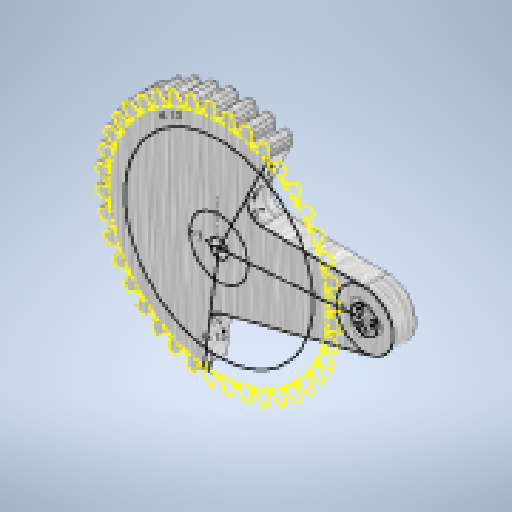
# Autodesk Inventor part: 最終段m2z40
Saved by Autodesk Inventor 2023 (Build 270158030, 158C)
## iProperties
Created: 2022-03-13
Part Number: 最終段m2z40
Material: アルミニウム 7075
Document SubType Name: Modeling
Designer: acps
Density: 2.81 g/cm^3
Appearance: サテン - ブラシ仕上げ 重厚
Author: acps
Autodesk Inventor part; units mm, degrees
(part 1 of 2)
ref_plane "YZ Plane" through (0, 0, 0) normal (1, 0, 0) x (0, 1, 0)
ref_plane "XZ Plane" through (0, 0, 0) normal (0, 1, 0) x (-1, 0, 0)
ref_plane "XY Plane" through (0, 0, 0) normal (0, 0, 1) x (1, 0, 0)
sketch "Sketch1" plane through (0, 0, 0) normal (0, 0, 1) x (1, 0, 0)
  arc A0 (0.9701, 39.1647) -> (0.7425, 38.3328) centre (9.8386, 36.2911) ccw
  arc A1 (1.4107, 40.3306) -> (0.9701, 39.1647) centre (13.2368, 35.1958) ccw
  arc A2 (2.1934, 41.9015) -> (1.4107, 40.3306) centre (16.718, 33.6843) ccw
  arc A3 (-5.1685, 38.8343) -> (-5.2632, 37.977) centre (4.0403, 37.3834) ccw
  arc A4 (-4.913, 40.0655) -> (-5.1685, 38.8343) centre (7.568, 36.8332) ccw
  arc A5 (-4.3885, 41.7288) -> (-4.913, 40.0655) centre (11.2428, 35.8848) ccw
  arc A6 (-11.1799, 37.5477) -> (-11.1393, 36.6861) centre (-1.8575, 37.5552) ccw
  arc A7 (-11.1212, 38.7926) -> (-11.1799, 37.5477) centre (1.7129, 37.5636) ccw
  arc A8 (-10.8623, 40.5285) -> (-11.1212, 38.7926) centre (5.4908, 37.2018) ccw
  arc A9 (-16.916, 35.3365) -> (-16.7411, 34.4919) centre (-7.7096, 36.8023) ccw
  arc A10 (-17.0535, 36.5863) -> (-16.916, 35.3365) centre (-4.1845, 37.3691) ccw
  arc A11 (-17.0686, 38.3303) -> (-17.0535, 36.5863) centre (-0.3965, 37.6027) ccw
  arc A12 (-22.2356, 32.2552) -> (-21.9307, 31.4483) centre (-13.3718, 35.1431) ccw
  arc A13 (-22.5669, 33.4681) -> (-22.2356, 32.2552) centre (-9.9788, 36.2544) ccw
  arc A14 (-22.8546, 35.1883) -> (-22.5669, 33.4681) centre (-6.2739, 37.0778) ccw
  arc A15 (-27.0076, 28.3796) -> (-26.5803, 27.6304) centre (-18.7048, 32.6187) ccw
  arc A16 (-27.5246, 29.5259) -> (-27.0076, 28.3796) centre (-15.5273, 34.247) ccw
  arc A17 (-28.0779, 31.1798) -> (-27.5246, 29.5259) centre (-11.9969, 35.6398) ccw
  arc A18 (-31.1147, 23.8053) -> (-30.5755, 23.1322) centre (-23.5772, 29.291) ccw
  arc A19 (-31.8046, 24.8565) -> (-31.1147, 23.8053) centre (-20.6936, 31.3964) ccw
  arc A20 (-32.6098, 26.4036) -> (-31.8046, 24.8565) centre (-17.4245, 33.3243) ccw
  arc A21 (-34.4556, 18.6448) -> (-33.8177, 18.0643) centre (-27.869, 25.2421) ccw
  arc A22 (-35.3014, 19.5752) -> (-34.4556, 18.6448) centre (-25.3503, 27.7726) ccw
  arc A23 (-36.3388, 20.9772) -> (-35.3014, 19.5752) centre (-22.4231, 30.1882) ccw
  arc A24 (-36.9365, 13.0169) -> (-36.2272, 12.5517) centre (-31.4746, 20.5717) ccw
  arc A25 (-37.9291, 13.8118) -> (-36.9365, 13.0169) centre (-29.3828, 23.4651) ccw
  arc A26 (-39.1729, 15.0343) -> (-37.9291, 13.8118) centre (-26.8695, 26.3088) ccw
  arc A27 (-38.5308, 7.0849) -> (-37.7447, 6.73) centre (-34.3052, 15.3947) ccw
  arc A28 (-39.6227, 7.7084) -> (-38.5308, 7.0849) centre (-32.6918, 18.5797) ccw
  arc A29 (-41.0425, 8.7212) -> (-39.6227, 7.7084) centre (-30.6543, 21.7816) ccw
  arc A30 (-39.1647, 0.9701) -> (-38.3328, 0.7425) centre (-36.2911, 9.8386) ccw
  arc A31 (-40.3306, 1.4107) -> (-39.1647, 0.9701) centre (-35.1958, 13.2368) ccw
  arc A32 (-41.9015, 2.1934) -> (-40.3306, 1.4107) centre (-33.6843, 16.718) ccw
  arc A33 (-38.8343, -5.1685) -> (-37.977, -5.2632) centre (-37.3834, 4.0403) ccw
  arc A34 (-40.0655, -4.913) -> (-38.8343, -5.1685) centre (-36.8332, 7.568) ccw
  arc A35 (-41.7288, -4.3885) -> (-40.0655, -4.913) centre (-35.8848, 11.2428) ccw
  arc A36 (-37.5477, -11.1799) -> (-36.6861, -11.1393) centre (-37.5552, -1.8575) ccw
  arc A37 (-38.7926, -11.1212) -> (-37.5477, -11.1799) centre (-37.5636, 1.7129) ccw
  arc A38 (-40.5285, -10.8623) -> (-38.7926, -11.1212) centre (-37.2018, 5.4908) ccw
  arc A39 (-35.3365, -16.916) -> (-34.4919, -16.7411) centre (-36.8023, -7.7096) ccw
  arc A40 (-36.5863, -17.0535) -> (-35.3365, -16.916) centre (-37.3691, -4.1845) ccw
  arc A41 (-38.3303, -17.0686) -> (-36.5863, -17.0535) centre (-37.6027, -0.3965) ccw
  arc A42 (-32.2552, -22.2356) -> (-31.4483, -21.9307) centre (-35.1431, -13.3718) ccw
  arc A43 (-33.4681, -22.5669) -> (-32.2552, -22.2356) centre (-36.2544, -9.9788) ccw
  arc A44 (-35.1883, -22.8546) -> (-33.4681, -22.5669) centre (-37.0778, -6.2739) ccw
  arc A45 (-28.3796, -27.0076) -> (-27.6304, -26.5803) centre (-32.6187, -18.7048) ccw
  arc A46 (-29.5259, -27.5246) -> (-28.3796, -27.0076) centre (-34.247, -15.5273) ccw
  arc A47 (-31.1798, -28.0779) -> (-29.5259, -27.5246) centre (-35.6398, -11.9969) ccw
  arc A48 (-23.8053, -31.1147) -> (-23.1322, -30.5754) centre (-29.291, -23.5771) ccw
  arc A49 (-24.8565, -31.8046) -> (-23.8053, -31.1147) centre (-31.3964, -20.6936) ccw
  arc A50 (-26.4036, -32.6098) -> (-24.8565, -31.8046) centre (-33.3243, -17.4245) ccw
  arc A51 (-18.6448, -34.4556) -> (-18.0643, -33.8177) centre (-25.2421, -27.869) ccw
  arc A52 (-19.5752, -35.3014) -> (-18.6448, -34.4556) centre (-27.7726, -25.3503) ccw
  arc A53 (-20.9772, -36.3388) -> (-19.5752, -35.3014) centre (-30.1882, -22.4231) ccw
  arc A54 (-13.0252, -36.9481) -> (-12.5517, -36.2272) centre (-20.5717, -31.4746) ccw
  arc A55 (-13.8118, -37.9291) -> (-13.0252, -36.9481) centre (-23.4651, -29.3828) ccw
  arc A56 (-15.0343, -39.1729) -> (-13.8118, -37.9291) centre (-26.3088, -26.8695) ccw
  arc A57 (-7.0849, -38.5308) -> (-6.73, -37.7447) centre (-15.3947, -34.3052) ccw
  arc A58 (-7.7084, -39.6227) -> (-7.0849, -38.5308) centre (-18.5797, -32.6918) ccw
  arc A59 (-8.7212, -41.0425) -> (-7.7084, -39.6227) centre (-21.7816, -30.6543) ccw
  arc A60 (-0.9701, -39.1647) -> (-0.7425, -38.3328) centre (-9.8386, -36.2911) ccw
  arc A61 (-1.4151, -40.3408) -> (-0.9701, -39.1647) centre (-13.2368, -35.1958) ccw
  arc A62 (-2.1934, -41.9015) -> (-1.4151, -40.3408) centre (-16.718, -33.6843) ccw
  arc A63 (5.1685, -38.8343) -> (5.2632, -37.977) centre (-4.0403, -37.3834) ccw
  arc A64 (4.913, -40.0655) -> (5.1685, -38.8343) centre (-7.568, -36.8332) ccw
  arc A65 (4.3885, -41.7288) -> (4.913, -40.0655) centre (-11.2428, -35.8848) ccw
  arc A66 (11.1799, -37.5477) -> (11.1393, -36.6861) centre (1.8575, -37.5552) ccw
  arc A67 (11.1201, -38.8036) -> (11.1799, -37.5477) centre (-1.7129, -37.5636) ccw
  arc A68 (10.8623, -40.5285) -> (11.1201, -38.8036) centre (-5.4908, -37.2018) ccw
  arc A69 (16.916, -35.3365) -> (16.7411, -34.4919) centre (7.7096, -36.8023) ccw
  arc A70 (17.0535, -36.5863) -> (16.916, -35.3365) centre (4.1845, -37.3691) ccw
  arc A71 (17.0686, -38.3303) -> (17.0535, -36.5863) centre (0.3965, -37.6027) ccw
  arc A72 (22.2356, -32.2552) -> (21.9307, -31.4483) centre (13.3718, -35.1431) ccw
  arc A73 (22.5669, -33.4681) -> (22.2356, -32.2552) centre (9.9788, -36.2544) ccw
  arc A74 (22.8546, -35.1883) -> (22.5669, -33.4681) centre (6.2739, -37.0778) ccw
  arc A75 (27.0076, -28.3796) -> (26.5803, -27.6304) centre (18.7048, -32.6187) ccw
  arc A76 (27.5246, -29.5259) -> (27.0076, -28.3796) centre (15.5273, -34.247) ccw
  arc A77 (28.0779, -31.1798) -> (27.5246, -29.5259) centre (11.9969, -35.6398) ccw
  arc A78 (31.1147, -23.8053) -> (30.5755, -23.1322) centre (23.5772, -29.291) ccw
  arc A79 (31.8046, -24.8565) -> (31.1147, -23.8053) centre (20.6936, -31.3964) ccw
  arc A80 (32.6098, -26.4036) -> (31.8046, -24.8565) centre (17.4245, -33.3243) ccw
  arc A81 (34.4556, -18.6448) -> (33.8177, -18.0643) centre (27.869, -25.2421) ccw
  arc A82 (35.3014, -19.5752) -> (34.4556, -18.6448) centre (25.3503, -27.7726) ccw
  arc A83 (36.3388, -20.9772) -> (35.3014, -19.5752) centre (22.4231, -30.1882) ccw
  arc A84 (36.9481, -13.0252) -> (36.2272, -12.5517) centre (31.4746, -20.5717) ccw
  arc A85 (37.9291, -13.8118) -> (36.9481, -13.0252) centre (29.3828, -23.4651) ccw
  arc A86 (39.1729, -15.0343) -> (37.9291, -13.8118) centre (26.8695, -26.3088) ccw
  arc A87 (38.5308, -7.0849) -> (37.7447, -6.73) centre (34.3052, -15.3947) ccw
  arc A88 (39.6227, -7.7084) -> (38.5308, -7.0849) centre (32.6918, -18.5797) ccw
  arc A89 (41.0425, -8.7212) -> (39.6227, -7.7084) centre (30.6543, -21.7816) ccw
  arc A90 (39.1647, -0.9701) -> (38.3328, -0.7425) centre (36.2911, -9.8386) ccw
  arc A91 (40.3408, -1.4151) -> (39.1647, -0.9701) centre (35.1958, -13.2368) ccw
  arc A92 (41.9015, -2.1934) -> (40.3408, -1.4151) centre (33.6843, -16.718) ccw
  arc A93 (38.8343, 5.1685) -> (37.977, 5.2632) centre (37.3834, -4.0403) ccw
  arc A94 (40.0655, 4.913) -> (38.8343, 5.1685) centre (36.8332, -7.568) ccw
  arc A95 (41.7288, 4.3885) -> (40.0655, 4.913) centre (35.8848, -11.2428) ccw
  arc A96 (37.5477, 11.1799) -> (36.6861, 11.1393) centre (37.5552, 1.8575) ccw
  arc A97 (38.8036, 11.1201) -> (37.5477, 11.1799) centre (37.5636, -1.7129) ccw
  arc A98 (40.5285, 10.8623) -> (38.8036, 11.1201) centre (37.2018, -5.4908) ccw
  arc A99 (35.3365, 16.916) -> (34.4919, 16.7411) centre (36.8023, 7.7096) ccw
  arc A100 (36.5863, 17.0535) -> (35.3365, 16.916) centre (37.3691, 4.1845) ccw
  arc A101 (38.3303, 17.0686) -> (36.5863, 17.0535) centre (37.6027, 0.3965) ccw
  arc A102 (32.2552, 22.2356) -> (31.4483, 21.9307) centre (35.1431, 13.3718) ccw
  arc A103 (33.4681, 22.5669) -> (32.2552, 22.2356) centre (36.2544, 9.9788) ccw
  arc A104 (35.1883, 22.8546) -> (33.4681, 22.5669) centre (37.0778, 6.2739) ccw
  arc A105 (28.3796, 27.0076) -> (27.6304, 26.5803) centre (32.6187, 18.7048) ccw
  arc A106 (29.5259, 27.5246) -> (28.3796, 27.0076) centre (34.247, 15.5273) ccw
  arc A107 (31.1798, 28.0779) -> (29.5259, 27.5246) centre (35.6398, 11.9969) ccw
  arc A108 (23.8053, 31.1147) -> (23.1322, 30.5755) centre (29.291, 23.5772) ccw
  arc A109 (24.8565, 31.8046) -> (23.8053, 31.1147) centre (31.3964, 20.6936) ccw
  arc A110 (26.4036, 32.6098) -> (24.8565, 31.8046) centre (33.3243, 17.4245) ccw
  arc A111 (18.6448, 34.4556) -> (18.0643, 33.8177) centre (25.2421, 27.869) ccw
  arc A112 (19.5752, 35.3014) -> (18.6448, 34.4556) centre (27.7726, 25.3503) ccw
  arc A113 (20.9772, 36.3388) -> (19.5752, 35.3014) centre (30.1882, 22.4231) ccw
  arc A114 (13.0252, 36.9481) -> (12.5517, 36.2272) centre (20.5717, 31.4746) ccw
  arc A115 (13.8118, 37.9291) -> (13.0252, 36.9481) centre (23.4651, 29.3828) ccw
  arc A116 (15.0343, 39.1729) -> (13.8118, 37.9291) centre (26.3088, 26.8695) ccw
  arc A117 (7.0849, 38.5308) -> (6.73, 37.7447) centre (15.3947, 34.3052) ccw
  arc A118 (7.7084, 39.6227) -> (7.0849, 38.5308) centre (18.5797, 32.6918) ccw
  arc A119 (8.7212, 41.0425) -> (7.7084, 39.6227) centre (21.7816, 30.6543) ccw
  arc A120 (-0.7425, 38.3328) -> (-0.9657, 39.1511) centre (-9.8386, 36.2911) ccw
  arc A121 (-0.9657, 39.1511) -> (-1.4151, 40.3408) centre (-13.2368, 35.1958) ccw
  arc A122 (-1.4151, 40.3408) -> (-2.1934, 41.9015) centre (-16.718, 33.6843) ccw
  arc A123 (-6.73, 37.7447) -> (-7.0849, 38.5308) centre (-15.3947, 34.3052) ccw
  arc A124 (-7.0849, 38.5308) -> (-7.7084, 39.6227) centre (-18.5797, 32.6918) ccw
  arc A125 (-7.7084, 39.6227) -> (-8.7212, 41.0425) centre (-21.7816, 30.6543) ccw
  arc A126 (-12.5517, 36.2272) -> (-13.0252, 36.9481) centre (-20.5717, 31.4746) ccw
  arc A127 (-13.0252, 36.9481) -> (-13.8118, 37.9291) centre (-23.4651, 29.3828) ccw
  arc A128 (-13.8118, 37.9291) -> (-15.0343, 39.1729) centre (-26.3088, 26.8695) ccw
  arc A129 (-18.0643, 33.8177) -> (-18.6448, 34.4556) centre (-25.2421, 27.869) ccw
  arc A130 (-18.6448, 34.4556) -> (-19.5752, 35.3014) centre (-27.7726, 25.3503) ccw
  arc A131 (-19.5752, 35.3014) -> (-20.9772, 36.3388) centre (-30.1882, 22.4231) ccw
  arc A132 (-23.1322, 30.5755) -> (-23.8053, 31.1147) centre (-29.291, 23.5772) ccw
  arc A133 (-23.8053, 31.1147) -> (-24.8565, 31.8046) centre (-31.3964, 20.6936) ccw
  arc A134 (-24.8565, 31.8046) -> (-26.4036, 32.6098) centre (-33.3243, 17.4245) ccw
  arc A135 (-27.6304, 26.5803) -> (-28.3796, 27.0076) centre (-32.6187, 18.7048) ccw
  arc A136 (-28.3796, 27.0076) -> (-29.5259, 27.5246) centre (-34.247, 15.5273) ccw
  arc A137 (-29.5259, 27.5246) -> (-31.1798, 28.0779) centre (-35.6398, 11.9969) ccw
  arc A138 (-31.4483, 21.9307) -> (-32.2552, 22.2356) centre (-35.1431, 13.3718) ccw
  arc A139 (-32.2552, 22.2356) -> (-33.4681, 22.5669) centre (-36.2544, 9.9788) ccw
  arc A140 (-33.4681, 22.5669) -> (-35.1883, 22.8546) centre (-37.0778, 6.2739) ccw
  arc A141 (-34.4919, 16.7411) -> (-35.3365, 16.916) centre (-36.8023, 7.7096) ccw
  arc A142 (-35.3365, 16.916) -> (-36.5863, 17.0535) centre (-37.3691, 4.1845) ccw
  arc A143 (-36.5863, 17.0535) -> (-38.3303, 17.0686) centre (-37.6027, 0.3965) ccw
  arc A144 (-36.6861, 11.1393) -> (-37.5477, 11.1799) centre (-37.5552, 1.8575) ccw
  arc A145 (-37.5477, 11.1799) -> (-38.8036, 11.1201) centre (-37.5636, -1.7129) ccw
  arc A146 (-38.8036, 11.1201) -> (-40.5285, 10.8623) centre (-37.2018, -5.4908) ccw
  arc A147 (-37.977, 5.2632) -> (-38.8343, 5.1685) centre (-37.3834, -4.0403) ccw
  arc A148 (-38.8343, 5.1685) -> (-40.0655, 4.913) centre (-36.8332, -7.568) ccw
  arc A149 (-40.0655, 4.913) -> (-41.7288, 4.3885) centre (-35.8848, -11.2428) ccw
  arc A150 (-38.3328, -0.7425) -> (-39.1647, -0.9701) centre (-36.2911, -9.8386) ccw
  arc A151 (-39.1647, -0.9701) -> (-40.3306, -1.4107) centre (-35.1958, -13.2368) ccw
  arc A152 (-40.3306, -1.4107) -> (-41.9015, -2.1934) centre (-33.6843, -16.718) ccw
  arc A153 (-37.7447, -6.73) -> (-38.5308, -7.0849) centre (-34.3052, -15.3947) ccw
  arc A154 (-38.5308, -7.0849) -> (-39.6227, -7.7084) centre (-32.6918, -18.5797) ccw
  arc A155 (-39.6227, -7.7084) -> (-41.0425, -8.7212) centre (-30.6543, -21.7816) ccw
  arc A156 (-36.2272, -12.5517) -> (-36.9481, -13.0252) centre (-31.4746, -20.5717) ccw
  arc A157 (-36.9481, -13.0252) -> (-37.9291, -13.8118) centre (-29.3828, -23.4651) ccw
  arc A158 (-37.9291, -13.8118) -> (-39.1729, -15.0343) centre (-26.8695, -26.3088) ccw
  arc A159 (-33.8177, -18.0643) -> (-34.4556, -18.6448) centre (-27.869, -25.2421) ccw
  arc A160 (-34.4556, -18.6448) -> (-35.3014, -19.5752) centre (-25.3503, -27.7726) ccw
  arc A161 (-35.3014, -19.5752) -> (-36.3388, -20.9772) centre (-22.4231, -30.1882) ccw
  arc A162 (-30.5754, -23.1322) -> (-31.1147, -23.8053) centre (-23.5771, -29.291) ccw
  arc A163 (-31.1147, -23.8053) -> (-31.8046, -24.8565) centre (-20.6936, -31.3964) ccw
  arc A164 (-31.8046, -24.8565) -> (-32.6098, -26.4036) centre (-17.4245, -33.3243) ccw
  arc A165 (-26.5803, -27.6304) -> (-27.0076, -28.3796) centre (-18.7048, -32.6187) ccw
  arc A166 (-27.0076, -28.3796) -> (-27.5246, -29.5259) centre (-15.5273, -34.247) ccw
  arc A167 (-27.5246, -29.5259) -> (-28.0779, -31.1798) centre (-11.9969, -35.6398) ccw
  arc A168 (-21.9307, -31.4483) -> (-22.2356, -32.2552) centre (-13.3718, -35.1431) ccw
  arc A169 (-22.2356, -32.2552) -> (-22.5669, -33.4681) centre (-9.9788, -36.2544) ccw
  arc A170 (-22.5669, -33.4681) -> (-22.8546, -35.1883) centre (-6.2739, -37.0778) ccw
  arc A171 (-16.7411, -34.4919) -> (-16.916, -35.3365) centre (-7.7096, -36.8023) ccw
  arc A172 (-16.916, -35.3365) -> (-17.0535, -36.5863) centre (-4.1845, -37.3691) ccw
  arc A173 (-17.0535, -36.5863) -> (-17.0686, -38.3303) centre (-0.3965, -37.6027) ccw
  arc A174 (-11.1393, -36.6861) -> (-11.1799, -37.5477) centre (-1.8575, -37.5552) ccw
  arc A175 (-11.1799, -37.5477) -> (-11.1201, -38.8036) centre (1.7129, -37.5636) ccw
  arc A176 (-11.1201, -38.8036) -> (-10.8623, -40.5285) centre (5.4908, -37.2018) ccw
  arc A177 (-5.2632, -37.977) -> (-5.1685, -38.8343) centre (4.0403, -37.3834) ccw
  arc A178 (-5.1685, -38.8343) -> (-4.913, -40.0655) centre (7.568, -36.8332) ccw
  arc A179 (-4.913, -40.0655) -> (-4.3885, -41.7288) centre (11.2428, -35.8848) ccw
  arc A180 (0.7425, -38.3328) -> (0.9701, -39.1647) centre (9.8386, -36.2911) ccw
  arc A181 (0.9701, -39.1647) -> (1.4151, -40.3408) centre (13.2368, -35.1958) ccw
  arc A182 (1.4151, -40.3408) -> (2.1934, -41.9015) centre (16.718, -33.6843) ccw
  arc A183 (6.73, -37.7447) -> (7.0849, -38.5308) centre (15.3947, -34.3052) ccw
  arc A184 (7.0849, -38.5308) -> (7.7084, -39.6227) centre (18.5797, -32.6918) ccw
  arc A185 (7.7084, -39.6227) -> (8.7212, -41.0425) centre (21.7816, -30.6543) ccw
  arc A186 (12.5517, -36.2272) -> (13.0252, -36.9481) centre (20.5717, -31.4746) ccw
  arc A187 (13.0252, -36.9481) -> (13.8118, -37.9291) centre (23.4651, -29.3828) ccw
  arc A188 (13.8118, -37.9291) -> (15.0343, -39.1729) centre (26.3088, -26.8695) ccw
  arc A189 (18.0643, -33.8177) -> (18.6448, -34.4556) centre (25.2421, -27.869) ccw
  arc A190 (18.6448, -34.4556) -> (19.5752, -35.3014) centre (27.7726, -25.3503) ccw
  arc A191 (19.5752, -35.3014) -> (20.9772, -36.3388) centre (30.1882, -22.4231) ccw
  arc A192 (23.1322, -30.5755) -> (23.8053, -31.1147) centre (29.291, -23.5772) ccw
  arc A193 (23.8053, -31.1147) -> (24.8565, -31.8046) centre (31.3964, -20.6936) ccw
  arc A194 (24.8565, -31.8046) -> (26.4036, -32.6098) centre (33.3243, -17.4245) ccw
  arc A195 (27.6304, -26.5803) -> (28.3796, -27.0076) centre (32.6187, -18.7048) ccw
  arc A196 (28.3796, -27.0076) -> (29.5259, -27.5246) centre (34.247, -15.5273) ccw
  arc A197 (29.5259, -27.5246) -> (31.1798, -28.0779) centre (35.6398, -11.9969) ccw
  arc A198 (31.4483, -21.9307) -> (32.2552, -22.2356) centre (35.1431, -13.3718) ccw
  arc A199 (32.2552, -22.2356) -> (33.4681, -22.5669) centre (36.2544, -9.9788) ccw
  arc A200 (33.4681, -22.5669) -> (35.1883, -22.8546) centre (37.0778, -6.2739) ccw
  arc A201 (34.4919, -16.7411) -> (35.3365, -16.916) centre (36.8023, -7.7096) ccw
  arc A202 (35.3365, -16.916) -> (36.5863, -17.0535) centre (37.3691, -4.1845) ccw
  arc A203 (36.5863, -17.0535) -> (38.3303, -17.0686) centre (37.6027, -0.3965) ccw
  arc A204 (36.6861, -11.1393) -> (37.5477, -11.1799) centre (37.5552, -1.8575) ccw
  arc A205 (37.5477, -11.1799) -> (38.8036, -11.1201) centre (37.5636, 1.7129) ccw
  arc A206 (38.8036, -11.1201) -> (40.5285, -10.8623) centre (37.2018, 5.4908) ccw
  arc A207 (37.977, -5.2632) -> (38.8343, -5.1685) centre (37.3834, 4.0403) ccw
  arc A208 (38.8343, -5.1685) -> (40.0655, -4.913) centre (36.8332, 7.568) ccw
  arc A209 (40.0655, -4.913) -> (41.7288, -4.3885) centre (35.8848, 11.2428) ccw
  arc A210 (38.3328, 0.7425) -> (39.1647, 0.9701) centre (36.2911, 9.8386) ccw
  arc A211 (39.1647, 0.9701) -> (40.3306, 1.4107) centre (35.1958, 13.2368) ccw
  arc A212 (40.3306, 1.4107) -> (41.9015, 2.1934) centre (33.6843, 16.718) ccw
  arc A213 (37.7447, 6.73) -> (38.5308, 7.0849) centre (34.3052, 15.3947) ccw
  arc A214 (38.5308, 7.0849) -> (39.6227, 7.7084) centre (32.6918, 18.5797) ccw
  arc A215 (39.6227, 7.7084) -> (41.0425, 8.7212) centre (30.6543, 21.7816) ccw
  arc A216 (36.2272, 12.5517) -> (36.9481, 13.0252) centre (31.4746, 20.5717) ccw
  arc A217 (36.9481, 13.0252) -> (37.9207, 13.8045) centre (29.3828, 23.4651) ccw
  arc A218 (37.9207, 13.8045) -> (39.1729, 15.0343) centre (26.8695, 26.3088) ccw
  arc A219 (33.8177, 18.0643) -> (34.4556, 18.6448) centre (27.869, 25.2421) ccw
  arc A220 (34.4556, 18.6448) -> (35.3014, 19.5752) centre (25.3503, 27.7726) ccw
  arc A221 (35.3014, 19.5752) -> (36.3388, 20.9772) centre (22.4231, 30.1882) ccw
  arc A222 (30.5755, 23.1322) -> (31.1147, 23.8053) centre (23.5772, 29.291) ccw
  arc A223 (31.1147, 23.8053) -> (31.8046, 24.8565) centre (20.6936, 31.3964) ccw
  arc A224 (31.8046, 24.8565) -> (32.6098, 26.4036) centre (17.4245, 33.3243) ccw
  arc A225 (26.5803, 27.6304) -> (27.0076, 28.3796) centre (18.7048, 32.6187) ccw
  arc A226 (27.0076, 28.3796) -> (27.5246, 29.5259) centre (15.5273, 34.247) ccw
  arc A227 (27.5246, 29.5259) -> (28.0779, 31.1798) centre (11.9969, 35.6398) ccw
  arc A228 (21.9307, 31.4483) -> (22.2356, 32.2552) centre (13.3718, 35.1431) ccw
  arc A229 (22.2356, 32.2552) -> (22.5669, 33.4681) centre (9.9788, 36.2544) ccw
  arc A230 (22.5669, 33.4681) -> (22.8546, 35.1883) centre (6.2739, 37.0778) ccw
  arc A231 (16.7411, 34.4919) -> (16.916, 35.3365) centre (7.7096, 36.8023) ccw
  arc A232 (16.916, 35.3365) -> (17.0535, 36.5863) centre (4.1845, 37.3691) ccw
  arc A233 (17.0535, 36.5863) -> (17.0686, 38.3303) centre (0.3965, 37.6027) ccw
  arc A234 (11.1393, 36.6861) -> (11.1799, 37.5477) centre (1.8575, 37.5552) ccw
  arc A235 (11.1799, 37.5477) -> (11.1201, 38.8036) centre (-1.7129, 37.5636) ccw
  arc A236 (11.1201, 38.8036) -> (10.8623, 40.5285) centre (-5.4908, 37.2018) ccw
  arc A237 (5.2632, 37.977) -> (5.1685, 38.8343) centre (-4.0403, 37.3834) ccw
  arc A238 (5.1685, 38.8343) -> (4.9158, 40.0547) centre (-7.568, 36.8332) ccw
  arc A239 (4.9158, 40.0547) -> (4.3885, 41.7288) centre (-11.2428, 35.8848) ccw
  arc A240 (0.7425, 38.3328) -> (-0.7425, 38.3328) centre (0, 0) ccw
  arc A241 (-5.2632, 37.977) -> (-6.73, 37.7447) centre (0, 0) ccw
  arc A242 (-11.1393, 36.6861) -> (-12.5517, 36.2272) centre (0, 0) ccw
  arc A243 (-16.7411, 34.4919) -> (-18.0643, 33.8177) centre (0, 0) ccw
  arc A244 (-21.9307, 31.4483) -> (-23.1322, 30.5755) centre (0, 0) ccw
  arc A245 (-26.5803, 27.6304) -> (-27.6304, 26.5803) centre (0, 0) ccw
  arc A246 (-30.5755, 23.1322) -> (-31.4483, 21.9307) centre (0, 0) ccw
  arc A247 (-33.8177, 18.0643) -> (-34.4919, 16.7411) centre (0, 0) ccw
  arc A248 (-36.2272, 12.5517) -> (-36.6861, 11.1393) centre (0, 0) ccw
  arc A249 (-37.7447, 6.73) -> (-37.977, 5.2632) centre (0, 0) ccw
  arc A250 (-38.3328, 0.7425) -> (-38.3328, -0.7425) centre (0, 0) ccw
  arc A251 (-37.977, -5.2632) -> (-37.7447, -6.73) centre (0, 0) ccw
  arc A252 (-36.6861, -11.1393) -> (-36.2272, -12.5517) centre (0, 0) ccw
  arc A253 (-34.4919, -16.7411) -> (-33.8177, -18.0643) centre (0, 0) ccw
  arc A254 (-31.4483, -21.9307) -> (-30.5754, -23.1322) centre (0, 0) ccw
  arc A255 (-27.6304, -26.5803) -> (-26.5803, -27.6304) centre (0, 0) ccw
  arc A256 (-23.1322, -30.5754) -> (-21.9307, -31.4483) centre (0, 0) ccw
  arc A257 (-18.0643, -33.8177) -> (-16.7411, -34.4919) centre (0, 0) ccw
  arc A258 (-12.5517, -36.2272) -> (-11.1393, -36.6861) centre (0, 0) ccw
  arc A259 (-6.73, -37.7447) -> (-5.2632, -37.977) centre (0, 0) ccw
  arc A260 (-0.7425, -38.3328) -> (0.7425, -38.3328) centre (0, 0) ccw
  arc A261 (5.2632, -37.977) -> (6.73, -37.7447) centre (0, 0) ccw
  arc A262 (11.1393, -36.6861) -> (12.5517, -36.2272) centre (0, 0) ccw
  arc A263 (16.7411, -34.4919) -> (18.0643, -33.8177) centre (0, 0) ccw
  arc A264 (21.9307, -31.4483) -> (23.1322, -30.5755) centre (0, 0) ccw
  arc A265 (26.5803, -27.6304) -> (27.6304, -26.5803) centre (0, 0) ccw
  arc A266 (30.5755, -23.1322) -> (31.4483, -21.9307) centre (0, 0) ccw
  arc A267 (33.8177, -18.0643) -> (34.4919, -16.7411) centre (0, 0) ccw
  arc A268 (36.2272, -12.5517) -> (36.6861, -11.1393) centre (0, 0) ccw
  arc A269 (37.7447, -6.73) -> (37.977, -5.2632) centre (0, 0) ccw
  arc A270 (38.3328, -0.7425) -> (38.3328, 0.7425) centre (0, 0) ccw
  arc A271 (37.977, 5.2632) -> (37.7447, 6.73) centre (0, 0) ccw
  arc A272 (36.6861, 11.1393) -> (36.2272, 12.5517) centre (0, 0) ccw
  arc A273 (34.4919, 16.7411) -> (33.8177, 18.0643) centre (0, 0) ccw
  arc A274 (31.4483, 21.9307) -> (30.5755, 23.1322) centre (0, 0) ccw
  arc A275 (27.6304, 26.5803) -> (26.5803, 27.6304) centre (0, 0) ccw
  arc A276 (23.1322, 30.5755) -> (21.9307, 31.4483) centre (0, 0) ccw
  arc A277 (18.0643, 33.8177) -> (16.7411, 34.4919) centre (0, 0) ccw
  arc A278 (12.5517, 36.2272) -> (11.1393, 36.6861) centre (0, 0) ccw
  arc A279 (6.73, 37.7447) -> (5.2632, 37.977) centre (0, 0) ccw
  arc A280 (-2.1934, 41.9015) -> (-4.3885, 41.7288) centre (0, 0) ccw
  arc A281 (-8.7212, 41.0425) -> (-10.8623, 40.5285) centre (0, 0) ccw
  arc A282 (-15.0343, 39.1729) -> (-17.0686, 38.3303) centre (0, 0) ccw
  arc A283 (-20.9772, 36.3388) -> (-22.8546, 35.1883) centre (0, 0) ccw
  arc A284 (-26.4036, 32.6098) -> (-28.0779, 31.1798) centre (0, 0) ccw
  arc A285 (-31.1798, 28.0779) -> (-32.6098, 26.4036) centre (0, 0) ccw
  arc A286 (-35.1883, 22.8546) -> (-36.3388, 20.9772) centre (0, 0) ccw
  arc A287 (-38.3303, 17.0686) -> (-39.1729, 15.0343) centre (0, 0) ccw
  arc A288 (-40.5285, 10.8623) -> (-41.0425, 8.7212) centre (0, 0) ccw
  arc A289 (-41.7288, 4.3885) -> (-41.9015, 2.1934) centre (0, 0) ccw
  arc A290 (-41.9015, -2.1934) -> (-41.7288, -4.3885) centre (0, 0) ccw
  arc A291 (-41.0425, -8.7212) -> (-40.5285, -10.8623) centre (0, 0) ccw
  arc A292 (-39.1729, -15.0343) -> (-38.3303, -17.0686) centre (0, 0) ccw
  arc A293 (-36.3388, -20.9772) -> (-35.1883, -22.8546) centre (0, 0) ccw
  arc A294 (-32.6098, -26.4036) -> (-31.1798, -28.0779) centre (0, 0) ccw
  arc A295 (-28.0779, -31.1798) -> (-26.4036, -32.6098) centre (0, 0) ccw
  arc A296 (-22.8546, -35.1883) -> (-20.9772, -36.3388) centre (0, 0) ccw
  arc A297 (-17.0686, -38.3303) -> (-15.0343, -39.1729) centre (0, 0) ccw
  arc A298 (-10.8623, -40.5285) -> (-8.7212, -41.0425) centre (0, 0) ccw
  arc A299 (-4.3885, -41.7288) -> (-2.1934, -41.9015) centre (0, 0) ccw
  arc A300 (2.1934, -41.9015) -> (4.3885, -41.7288) centre (0, 0) ccw
  arc A301 (8.7212, -41.0425) -> (10.8623, -40.5285) centre (0, 0) ccw
  arc A302 (15.0343, -39.1729) -> (17.0686, -38.3303) centre (0, 0) ccw
  arc A303 (20.9772, -36.3388) -> (22.8546, -35.1883) centre (0, 0) ccw
  arc A304 (26.4036, -32.6098) -> (28.0779, -31.1798) centre (0, 0) ccw
  arc A305 (31.1798, -28.0779) -> (32.6098, -26.4036) centre (0, 0) ccw
  arc A306 (35.1883, -22.8546) -> (36.3388, -20.9772) centre (0, 0) ccw
  arc A307 (38.3303, -17.0686) -> (39.1729, -15.0343) centre (0, 0) ccw
  arc A308 (40.5285, -10.8623) -> (41.0425, -8.7212) centre (0, 0) ccw
  arc A309 (41.7288, -4.3885) -> (41.9015, -2.1934) centre (0, 0) ccw
  arc A310 (41.9015, 2.1934) -> (41.7288, 4.3885) centre (0, 0) ccw
  arc A311 (41.0425, 8.7212) -> (40.5285, 10.8623) centre (0, 0) ccw
  arc A312 (39.1729, 15.0343) -> (38.3303, 17.0686) centre (0, 0) ccw
  arc A313 (36.3388, 20.9772) -> (35.1883, 22.8546) centre (0, 0) ccw
  arc A314 (32.6098, 26.4036) -> (31.1798, 28.0779) centre (0, 0) ccw
  arc A315 (28.0779, 31.1798) -> (26.4036, 32.6098) centre (0, 0) ccw
  arc A316 (22.8546, 35.1883) -> (20.9772, 36.3388) centre (0, 0) ccw
  arc A317 (17.0686, 38.3303) -> (15.0343, 39.1729) centre (0, 0) ccw
  arc A318 (10.8623, 40.5285) -> (8.7212, 41.0425) centre (0, 0) ccw
  arc A319 (4.3885, 41.7288) -> (2.1934, 41.9015) centre (0, 0) ccw
  point P0 (0, 0)
  constraints: 480 point on circle, 240 centre point, 2 horizontal alignment, 2 vertical alignment, 236 other
extrude "Extrusion1" add sketch "Sketch1" against normal blind 8
sketch "Sketch2" plane through (0, 0, 0) normal (0, 0, 1) x (1, 0, 0)
  circle A0 centre (0, 0) radius 3
  circle A1 centre (0, 0) radius 32.21
  arc A2 (-16.7411, 34.4919) -> (-18.0643, 33.8177) centre (0, 0) ccw projected
  circle A3 centre (0, 0) radius 10
  line L0 (0, 0) -> (0, 15.2394) construction
  arc A4 (37.977, 5.2632) -> (37.7447, 6.73) centre (0, 0) ccw projected
  arc A5 (0.7425, 38.3328) -> (-0.7425, 38.3328) centre (0, 0) ccw projected
  arc A6 (-0.7425, 38.3328) -> (-0.9657, 39.1511) centre (-9.8386, 36.2911) ccw projected
  arc A7 (-0.9657, 39.1511) -> (-1.4151, 40.3408) centre (-13.2368, 35.1958) ccw projected
  arc A8 (-1.4151, 40.3408) -> (-2.1934, 41.9015) centre (-16.718, 33.6843) ccw projected
  arc A9 (-2.1934, 41.9015) -> (-4.3885, 41.7288) centre (0, 0) ccw projected
  arc A10 (-4.3885, 41.7288) -> (-4.913, 40.0655) centre (11.2428, 35.8848) ccw projected
  arc A11 (-4.913, 40.0655) -> (-5.1685, 38.8343) centre (7.568, 36.8332) ccw projected
  arc A12 (-5.1685, 38.8343) -> (-5.2632, 37.977) centre (4.0403, 37.3834) ccw projected
  arc A13 (-5.2632, 37.977) -> (-6.73, 37.7447) centre (0, 0) ccw projected
  arc A14 (-6.73, 37.7447) -> (-7.0849, 38.5308) centre (-15.3947, 34.3052) ccw projected
  arc A15 (-7.0849, 38.5308) -> (-7.7084, 39.6227) centre (-18.5797, 32.6918) ccw projected
  arc A16 (-7.7084, 39.6227) -> (-8.7212, 41.0425) centre (-21.7816, 30.6543) ccw projected
  arc A17 (-8.7212, 41.0425) -> (-10.8623, 40.5285) centre (0, 0) ccw projected
  arc A18 (-10.8623, 40.5285) -> (-11.1212, 38.7926) centre (5.4908, 37.2018) ccw projected
  arc A19 (-11.1212, 38.7926) -> (-11.1799, 37.5477) centre (1.7129, 37.5636) ccw projected
  arc A20 (-11.1799, 37.5477) -> (-11.1393, 36.6861) centre (-1.8575, 37.5552) ccw projected
  arc A21 (-11.1393, 36.6861) -> (-12.5517, 36.2272) centre (0, 0) ccw projected
  arc A22 (-12.5517, 36.2272) -> (-13.0252, 36.9481) centre (-20.5717, 31.4746) ccw projected
  arc A23 (-13.0252, 36.9481) -> (-13.8118, 37.9291) centre (-23.4651, 29.3828) ccw projected
  arc A24 (-13.8118, 37.9291) -> (-15.0343, 39.1729) centre (-26.3088, 26.8695) ccw projected
  arc A25 (-15.0343, 39.1729) -> (-17.0686, 38.3303) centre (0, 0) ccw projected
  arc A26 (-17.0686, 38.3303) -> (-17.0535, 36.5863) centre (-0.3965, 37.6027) ccw projected
  arc A27 (-17.0535, 36.5863) -> (-16.916, 35.3365) centre (-4.1845, 37.3691) ccw projected
  arc A28 (-16.916, 35.3365) -> (-16.7411, 34.4919) centre (-7.7096, 36.8023) ccw projected
  arc A29 (-16.7411, 34.4919) -> (-18.0643, 33.8177) centre (0, 0) ccw projected
  arc A30 (-18.0643, 33.8177) -> (-18.6448, 34.4556) centre (-25.2421, 27.869) ccw projected
  arc A31 (-18.6448, 34.4556) -> (-19.5752, 35.3014) centre (-27.7726, 25.3503) ccw projected
  arc A32 (-19.5752, 35.3014) -> (-20.9772, 36.3388) centre (-30.1882, 22.4231) ccw projected
  arc A33 (-20.9772, 36.3388) -> (-22.8546, 35.1883) centre (0, 0) ccw projected
  arc A34 (-22.8546, 35.1883) -> (-22.5669, 33.4681) centre (-6.2739, 37.0778) ccw projected
  arc A35 (-22.5669, 33.4681) -> (-22.2356, 32.2552) centre (-9.9788, 36.2544) ccw projected
  arc A36 (-22.2356, 32.2552) -> (-21.9307, 31.4483) centre (-13.3718, 35.1431) ccw projected
  arc A37 (-21.9307, 31.4483) -> (-23.1322, 30.5755) centre (0, 0) ccw projected
  arc A38 (-23.1322, 30.5755) -> (-23.8053, 31.1147) centre (-29.291, 23.5772) ccw projected
  arc A39 (-23.8053, 31.1147) -> (-24.8565, 31.8046) centre (-31.3964, 20.6936) ccw projected
  arc A40 (-24.8565, 31.8046) -> (-26.4036, 32.6098) centre (-33.3243, 17.4245) ccw projected
  arc A41 (-26.4036, 32.6098) -> (-28.0779, 31.1798) centre (0, 0) ccw projected
  arc A42 (-28.0779, 31.1798) -> (-27.5246, 29.5259) centre (-11.9969, 35.6398) ccw projected
  arc A43 (-27.5246, 29.5259) -> (-27.0076, 28.3796) centre (-15.5273, 34.247) ccw projected
  arc A44 (-27.0076, 28.3796) -> (-26.5803, 27.6304) centre (-18.7048, 32.6187) ccw projected
  arc A45 (-26.5803, 27.6304) -> (-27.6304, 26.5803) centre (0, 0) ccw projected
  arc A46 (-27.6304, 26.5803) -> (-28.3796, 27.0076) centre (-32.6187, 18.7048) ccw projected
  arc A47 (-28.3796, 27.0076) -> (-29.5259, 27.5246) centre (-34.247, 15.5273) ccw projected
  arc A48 (-29.5259, 27.5246) -> (-31.1798, 28.0779) centre (-35.6398, 11.9969) ccw projected
  arc A49 (-31.1798, 28.0779) -> (-32.6098, 26.4036) centre (0, 0) ccw projected
  arc A50 (-32.6098, 26.4036) -> (-31.8046, 24.8565) centre (-17.4245, 33.3243) ccw projected
  arc A51 (-31.8046, 24.8565) -> (-31.1147, 23.8053) centre (-20.6936, 31.3964) ccw projected
  arc A52 (-31.1147, 23.8053) -> (-30.5755, 23.1322) centre (-23.5772, 29.291) ccw projected
  arc A53 (-30.5755, 23.1322) -> (-31.4483, 21.9307) centre (0, 0) ccw projected
  arc A54 (-31.4483, 21.9307) -> (-32.2552, 22.2356) centre (-35.1431, 13.3718) ccw projected
  arc A55 (-32.2552, 22.2356) -> (-33.4681, 22.5669) centre (-36.2544, 9.9788) ccw projected
  arc A56 (-33.4681, 22.5669) -> (-35.1883, 22.8546) centre (-37.0778, 6.2739) ccw projected
  arc A57 (-35.1883, 22.8546) -> (-36.3388, 20.9772) centre (0, 0) ccw projected
  arc A58 (-36.3388, 20.9772) -> (-35.3014, 19.5752) centre (-22.4231, 30.1882) ccw projected
  arc A59 (-35.3014, 19.5752) -> (-34.4556, 18.6448) centre (-25.3503, 27.7726) ccw projected
  arc A60 (-34.4556, 18.6448) -> (-33.8177, 18.0643) centre (-27.869, 25.2421) ccw projected
  arc A61 (-33.8177, 18.0643) -> (-34.4919, 16.7411) centre (0, 0) ccw projected
  arc A62 (-34.4919, 16.7411) -> (-35.3365, 16.916) centre (-36.8023, 7.7096) ccw projected
  arc A63 (-35.3365, 16.916) -> (-36.5863, 17.0535) centre (-37.3691, 4.1845) ccw projected
  arc A64 (-36.5863, 17.0535) -> (-38.3303, 17.0686) centre (-37.6027, 0.3965) ccw projected
  arc A65 (-38.3303, 17.0686) -> (-39.1729, 15.0343) centre (0, 0) ccw projected
  arc A66 (-39.1729, 15.0343) -> (-37.9291, 13.8118) centre (-26.8695, 26.3088) ccw projected
  arc A67 (-37.9291, 13.8118) -> (-36.9365, 13.0169) centre (-29.3828, 23.4651) ccw projected
  arc A68 (-36.9365, 13.0169) -> (-36.2272, 12.5517) centre (-31.4746, 20.5717) ccw projected
  arc A69 (-36.2272, 12.5517) -> (-36.6861, 11.1393) centre (0, 0) ccw projected
  arc A70 (-36.6861, 11.1393) -> (-37.5477, 11.1799) centre (-37.5552, 1.8575) ccw projected
  arc A71 (-37.5477, 11.1799) -> (-38.8036, 11.1201) centre (-37.5636, -1.7129) ccw projected
  arc A72 (-38.8036, 11.1201) -> (-40.5285, 10.8623) centre (-37.2018, -5.4908) ccw projected
  arc A73 (-40.5285, 10.8623) -> (-41.0425, 8.7212) centre (0, 0) ccw projected
  arc A74 (-41.0425, 8.7212) -> (-39.6227, 7.7084) centre (-30.6543, 21.7816) ccw projected
  arc A75 (-39.6227, 7.7084) -> (-38.5308, 7.0849) centre (-32.6918, 18.5797) ccw projected
  arc A76 (-38.5308, 7.0849) -> (-37.7447, 6.73) centre (-34.3052, 15.3947) ccw projected
  arc A77 (-37.7447, 6.73) -> (-37.977, 5.2632) centre (0, 0) ccw projected
  arc A78 (-37.977, 5.2632) -> (-38.8343, 5.1685) centre (-37.3834, -4.0403) ccw projected
  arc A79 (-38.8343, 5.1685) -> (-40.0655, 4.913) centre (-36.8332, -7.568) ccw projected
  arc A80 (-40.0655, 4.913) -> (-41.7288, 4.3885) centre (-35.8848, -11.2428) ccw projected
  arc A81 (-41.7288, 4.3885) -> (-41.9015, 2.1934) centre (0, 0) ccw projected
  arc A82 (-41.9015, 2.1934) -> (-40.3306, 1.4107) centre (-33.6843, 16.718) ccw projected
  arc A83 (-40.3306, 1.4107) -> (-39.1647, 0.9701) centre (-35.1958, 13.2368) ccw projected
  arc A84 (-39.1647, 0.9701) -> (-38.3328, 0.7425) centre (-36.2911, 9.8386) ccw projected
  arc A85 (-38.3328, 0.7425) -> (-38.3328, -0.7425) centre (0, 0) ccw projected
  arc A86 (-38.3328, -0.7425) -> (-39.1647, -0.9701) centre (-36.2911, -9.8386) ccw projected
  arc A87 (-39.1647, -0.9701) -> (-40.3306, -1.4107) centre (-35.1958, -13.2368) ccw projected
  arc A88 (-40.3306, -1.4107) -> (-41.9015, -2.1934) centre (-33.6843, -16.718) ccw projected
  arc A89 (-41.9015, -2.1934) -> (-41.7288, -4.3885) centre (0, 0) ccw projected
  arc A90 (-41.7288, -4.3885) -> (-40.0655, -4.913) centre (-35.8848, 11.2428) ccw projected
  arc A91 (-40.0655, -4.913) -> (-38.8343, -5.1685) centre (-36.8332, 7.568) ccw projected
  arc A92 (-38.8343, -5.1685) -> (-37.977, -5.2632) centre (-37.3834, 4.0403) ccw projected
  arc A93 (-37.977, -5.2632) -> (-37.7447, -6.73) centre (0, 0) ccw projected
  arc A94 (-37.7447, -6.73) -> (-38.5308, -7.0849) centre (-34.3052, -15.3947) ccw projected
  arc A95 (-38.5308, -7.0849) -> (-39.6227, -7.7084) centre (-32.6918, -18.5797) ccw projected
  arc A96 (-39.6227, -7.7084) -> (-41.0425, -8.7212) centre (-30.6543, -21.7816) ccw projected
  arc A97 (-41.0425, -8.7212) -> (-40.5285, -10.8623) centre (0, 0) ccw projected
  arc A98 (-40.5285, -10.8623) -> (-38.7926, -11.1212) centre (-37.2018, 5.4908) ccw projected
  arc A99 (-38.7926, -11.1212) -> (-37.5477, -11.1799) centre (-37.5636, 1.7129) ccw projected
  arc A100 (-37.5477, -11.1799) -> (-36.6861, -11.1393) centre (-37.5552, -1.8575) ccw projected
  arc A101 (-36.6861, -11.1393) -> (-36.2272, -12.5517) centre (0, 0) ccw projected
  arc A102 (-36.2272, -12.5517) -> (-36.9481, -13.0252) centre (-31.4746, -20.5717) ccw projected
  arc A103 (-36.9481, -13.0252) -> (-37.9291, -13.8118) centre (-29.3828, -23.4651) ccw projected
  arc A104 (-37.9291, -13.8118) -> (-39.1729, -15.0343) centre (-26.8695, -26.3088) ccw projected
  arc A105 (-39.1729, -15.0343) -> (-38.3303, -17.0686) centre (0, 0) ccw projected
  arc A106 (-38.3303, -17.0686) -> (-36.5863, -17.0535) centre (-37.6027, -0.3965) ccw projected
  arc A107 (-36.5863, -17.0535) -> (-35.3365, -16.916) centre (-37.3691, -4.1845) ccw projected
  arc A108 (-35.3365, -16.916) -> (-34.4919, -16.7411) centre (-36.8023, -7.7096) ccw projected
  arc A109 (-34.4919, -16.7411) -> (-33.8177, -18.0643) centre (0, 0) ccw projected
  arc A110 (-33.8177, -18.0643) -> (-34.4556, -18.6448) centre (-27.869, -25.2421) ccw projected
  arc A111 (-34.4556, -18.6448) -> (-35.3014, -19.5752) centre (-25.3503, -27.7726) ccw projected
  arc A112 (-35.3014, -19.5752) -> (-36.3388, -20.9772) centre (-22.4231, -30.1882) ccw projected
  arc A113 (-36.3388, -20.9772) -> (-35.1883, -22.8546) centre (0, 0) ccw projected
  arc A114 (-35.1883, -22.8546) -> (-33.4681, -22.5669) centre (-37.0778, -6.2739) ccw projected
  arc A115 (-33.4681, -22.5669) -> (-32.2552, -22.2356) centre (-36.2544, -9.9788) ccw projected
  arc A116 (-32.2552, -22.2356) -> (-31.4483, -21.9307) centre (-35.1431, -13.3718) ccw projected
  arc A117 (-31.4483, -21.9307) -> (-30.5754, -23.1322) centre (0, 0) ccw projected
  arc A118 (-30.5754, -23.1322) -> (-31.1147, -23.8053) centre (-23.5771, -29.291) ccw projected
  arc A119 (-31.1147, -23.8053) -> (-31.8046, -24.8565) centre (-20.6936, -31.3964) ccw projected
  arc A120 (-31.8046, -24.8565) -> (-32.6098, -26.4036) centre (-17.4245, -33.3243) ccw projected
  arc A121 (-32.6098, -26.4036) -> (-31.1798, -28.0779) centre (0, 0) ccw projected
  arc A122 (-31.1798, -28.0779) -> (-29.5259, -27.5246) centre (-35.6398, -11.9969) ccw projected
  arc A123 (-29.5259, -27.5246) -> (-28.3796, -27.0076) centre (-34.247, -15.5273) ccw projected
  arc A124 (-28.3796, -27.0076) -> (-27.6304, -26.5803) centre (-32.6187, -18.7048) ccw projected
  arc A125 (-27.6304, -26.5803) -> (-26.5803, -27.6304) centre (0, 0) ccw projected
  arc A126 (-26.5803, -27.6304) -> (-27.0076, -28.3796) centre (-18.7048, -32.6187) ccw projected
  arc A127 (-27.0076, -28.3796) -> (-27.5246, -29.5259) centre (-15.5273, -34.247) ccw projected
  arc A128 (-27.5246, -29.5259) -> (-28.0779, -31.1798) centre (-11.9969, -35.6398) ccw projected
  arc A129 (-28.0779, -31.1798) -> (-26.4036, -32.6098) centre (0, 0) ccw projected
  arc A130 (-26.4036, -32.6098) -> (-24.8565, -31.8046) centre (-33.3243, -17.4245) ccw projected
  arc A131 (-24.8565, -31.8046) -> (-23.8053, -31.1147) centre (-31.3964, -20.6936) ccw projected
  arc A132 (-23.8053, -31.1147) -> (-23.1322, -30.5754) centre (-29.291, -23.5771) ccw projected
  arc A133 (-23.1322, -30.5754) -> (-21.9307, -31.4483) centre (0, 0) ccw projected
  arc A134 (-21.9307, -31.4483) -> (-22.2356, -32.2552) centre (-13.3718, -35.1431) ccw projected
  arc A135 (-22.2356, -32.2552) -> (-22.5669, -33.4681) centre (-9.9788, -36.2544) ccw projected
  arc A136 (-22.5669, -33.4681) -> (-22.8546, -35.1883) centre (-6.2739, -37.0778) ccw projected
  arc A137 (-22.8546, -35.1883) -> (-20.9772, -36.3388) centre (0, 0) ccw projected
  arc A138 (-20.9772, -36.3388) -> (-19.5752, -35.3014) centre (-30.1882, -22.4231) ccw projected
  arc A139 (-19.5752, -35.3014) -> (-18.6448, -34.4556) centre (-27.7726, -25.3503) ccw projected
  arc A140 (-18.6448, -34.4556) -> (-18.0643, -33.8177) centre (-25.2421, -27.869) ccw projected
  arc A141 (-18.0643, -33.8177) -> (-16.7411, -34.4919) centre (0, 0) ccw projected
  arc A142 (-16.7411, -34.4919) -> (-16.916, -35.3365) centre (-7.7096, -36.8023) ccw projected
  arc A143 (-16.916, -35.3365) -> (-17.0535, -36.5863) centre (-4.1845, -37.3691) ccw projected
  arc A144 (-17.0535, -36.5863) -> (-17.0686, -38.3303) centre (-0.3965, -37.6027) ccw projected
  arc A145 (-17.0686, -38.3303) -> (-15.0343, -39.1729) centre (0, 0) ccw projected
  arc A146 (-15.0343, -39.1729) -> (-13.8118, -37.9291) centre (-26.3088, -26.8695) ccw projected
  arc A147 (-13.8118, -37.9291) -> (-13.0252, -36.9481) centre (-23.4651, -29.3828) ccw projected
  arc A148 (-13.0252, -36.9481) -> (-12.5517, -36.2272) centre (-20.5717, -31.4746) ccw projected
  arc A149 (-12.5517, -36.2272) -> (-11.1393, -36.6861) centre (0, 0) ccw projected
  arc A150 (-11.1393, -36.6861) -> (-11.1799, -37.5477) centre (-1.8575, -37.5552) ccw projected
  arc A151 (-11.1799, -37.5477) -> (-11.1201, -38.8036) centre (1.7129, -37.5636) ccw projected
  arc A152 (-11.1201, -38.8036) -> (-10.8623, -40.5285) centre (5.4908, -37.2018) ccw projected
  arc A153 (-10.8623, -40.5285) -> (-8.7212, -41.0425) centre (0, 0) ccw projected
  arc A154 (-8.7212, -41.0425) -> (-7.7084, -39.6227) centre (-21.7816, -30.6543) ccw projected
  arc A155 (-7.7084, -39.6227) -> (-7.0849, -38.5308) centre (-18.5797, -32.6918) ccw projected
  arc A156 (-7.0849, -38.5308) -> (-6.73, -37.7447) centre (-15.3947, -34.3052) ccw projected
  arc A157 (-6.73, -37.7447) -> (-5.2632, -37.977) centre (0, 0) ccw projected
  arc A158 (-5.2632, -37.977) -> (-5.1685, -38.8343) centre (4.0403, -37.3834) ccw projected
  arc A159 (-5.1685, -38.8343) -> (-4.913, -40.0655) centre (7.568, -36.8332) ccw projected
  arc A160 (-4.913, -40.0655) -> (-4.3885, -41.7288) centre (11.2428, -35.8848) ccw projected
  arc A161 (-4.3885, -41.7288) -> (-2.1934, -41.9015) centre (0, 0) ccw projected
  arc A162 (-2.1934, -41.9015) -> (-1.4151, -40.3408) centre (-16.718, -33.6843) ccw projected
  arc A163 (-1.4151, -40.3408) -> (-0.9701, -39.1647) centre (-13.2368, -35.1958) ccw projected
  arc A164 (-0.9701, -39.1647) -> (-0.7425, -38.3328) centre (-9.8386, -36.2911) ccw projected
  arc A165 (-0.7425, -38.3328) -> (0.7425, -38.3328) centre (0, 0) ccw projected
  arc A166 (0.7425, -38.3328) -> (0.9701, -39.1647) centre (9.8386, -36.2911) ccw projected
  arc A167 (0.9701, -39.1647) -> (1.4151, -40.3408) centre (13.2368, -35.1958) ccw projected
  arc A168 (1.4151, -40.3408) -> (2.1934, -41.9015) centre (16.718, -33.6843) ccw projected
  arc A169 (2.1934, -41.9015) -> (4.3885, -41.7288) centre (0, 0) ccw projected
  arc A170 (4.3885, -41.7288) -> (4.913, -40.0655) centre (-11.2428, -35.8848) ccw projected
  arc A171 (4.913, -40.0655) -> (5.1685, -38.8343) centre (-7.568, -36.8332) ccw projected
  arc A172 (5.1685, -38.8343) -> (5.2632, -37.977) centre (-4.0403, -37.3834) ccw projected
  arc A173 (5.2632, -37.977) -> (6.73, -37.7447) centre (0, 0) ccw projected
  arc A174 (6.73, -37.7447) -> (7.0849, -38.5308) centre (15.3947, -34.3052) ccw projected
  arc A175 (7.0849, -38.5308) -> (7.7084, -39.6227) centre (18.5797, -32.6918) ccw projected
  arc A176 (7.7084, -39.6227) -> (8.7212, -41.0425) centre (21.7816, -30.6543) ccw projected
  arc A177 (8.7212, -41.0425) -> (10.8623, -40.5285) centre (0, 0) ccw projected
  arc A178 (10.8623, -40.5285) -> (11.1201, -38.8036) centre (-5.4908, -37.2018) ccw projected
  arc A179 (11.1201, -38.8036) -> (11.1799, -37.5477) centre (-1.7129, -37.5636) ccw projected
  arc A180 (11.1799, -37.5477) -> (11.1393, -36.6861) centre (1.8575, -37.5552) ccw projected
  arc A181 (11.1393, -36.6861) -> (12.5517, -36.2272) centre (0, 0) ccw projected
  arc A182 (12.5517, -36.2272) -> (13.0252, -36.9481) centre (20.5717, -31.4746) ccw projected
  arc A183 (13.0252, -36.9481) -> (13.8118, -37.9291) centre (23.4651, -29.3828) ccw projected
  arc A184 (13.8118, -37.9291) -> (15.0343, -39.1729) centre (26.3088, -26.8695) ccw projected
  arc A185 (15.0343, -39.1729) -> (17.0686, -38.3303) centre (0, 0) ccw projected
  arc A186 (17.0686, -38.3303) -> (17.0535, -36.5863) centre (0.3965, -37.6027) ccw projected
  arc A187 (17.0535, -36.5863) -> (16.916, -35.3365) centre (4.1845, -37.3691) ccw projected
  arc A188 (16.916, -35.3365) -> (16.7411, -34.4919) centre (7.7096, -36.8023) ccw projected
  arc A189 (16.7411, -34.4919) -> (18.0643, -33.8177) centre (0, 0) ccw projected
  arc A190 (18.0643, -33.8177) -> (18.6448, -34.4556) centre (25.2421, -27.869) ccw projected
  arc A191 (18.6448, -34.4556) -> (19.5752, -35.3014) centre (27.7726, -25.3503) ccw projected
  arc A192 (19.5752, -35.3014) -> (20.9772, -36.3388) centre (30.1882, -22.4231) ccw projected
  arc A193 (20.9772, -36.3388) -> (22.8546, -35.1883) centre (0, 0) ccw projected
  arc A194 (22.8546, -35.1883) -> (22.5669, -33.4681) centre (6.2739, -37.0778) ccw projected
  arc A195 (22.5669, -33.4681) -> (22.2356, -32.2552) centre (9.9788, -36.2544) ccw projected
  arc A196 (22.2356, -32.2552) -> (21.9307, -31.4483) centre (13.3718, -35.1431) ccw projected
  arc A197 (21.9307, -31.4483) -> (23.1322, -30.5755) centre (0, 0) ccw projected
  arc A198 (23.1322, -30.5755) -> (23.8053, -31.1147) centre (29.291, -23.5772) ccw projected
  arc A199 (23.8053, -31.1147) -> (24.8565, -31.8046) centre (31.3964, -20.6936) ccw projected
  arc A200 (24.8565, -31.8046) -> (26.4036, -32.6098) centre (33.3243, -17.4245) ccw projected
  arc A201 (26.4036, -32.6098) -> (28.0779, -31.1798) centre (0, 0) ccw projected
  arc A202 (28.0779, -31.1798) -> (27.5246, -29.5259) centre (11.9969, -35.6398) ccw projected
  arc A203 (27.5246, -29.5259) -> (27.0076, -28.3796) centre (15.5273, -34.247) ccw projected
  arc A204 (27.0076, -28.3796) -> (26.5803, -27.6304) centre (18.7048, -32.6187) ccw projected
  arc A205 (26.5803, -27.6304) -> (27.6304, -26.5803) centre (0, 0) ccw projected
  arc A206 (27.6304, -26.5803) -> (28.3796, -27.0076) centre (32.6187, -18.7048) ccw projected
  arc A207 (28.3796, -27.0076) -> (29.5259, -27.5246) centre (34.247, -15.5273) ccw projected
  arc A208 (29.5259, -27.5246) -> (31.1798, -28.0779) centre (35.6398, -11.9969) ccw projected
  arc A209 (31.1798, -28.0779) -> (32.6098, -26.4036) centre (0, 0) ccw projected
  arc A210 (32.6098, -26.4036) -> (31.8046, -24.8565) centre (17.4245, -33.3243) ccw projected
  arc A211 (31.8046, -24.8565) -> (31.1147, -23.8053) centre (20.6936, -31.3964) ccw projected
  arc A212 (31.1147, -23.8053) -> (30.5755, -23.1322) centre (23.5772, -29.291) ccw projected
  arc A213 (30.5755, -23.1322) -> (31.4483, -21.9307) centre (0, 0) ccw projected
  arc A214 (31.4483, -21.9307) -> (32.2552, -22.2356) centre (35.1431, -13.3718) ccw projected
  arc A215 (32.2552, -22.2356) -> (33.4681, -22.5669) centre (36.2544, -9.9788) ccw projected
  arc A216 (33.4681, -22.5669) -> (35.1883, -22.8546) centre (37.0778, -6.2739) ccw projected
  arc A217 (35.1883, -22.8546) -> (36.3388, -20.9772) centre (0, 0) ccw projected
  arc A218 (36.3388, -20.9772) -> (35.3014, -19.5752) centre (22.4231, -30.1882) ccw projected
  arc A219 (35.3014, -19.5752) -> (34.4556, -18.6448) centre (25.3503, -27.7726) ccw projected
  arc A220 (34.4556, -18.6448) -> (33.8177, -18.0643) centre (27.869, -25.2421) ccw projected
  arc A221 (33.8177, -18.0643) -> (34.4919, -16.7411) centre (0, 0) ccw projected
  arc A222 (34.4919, -16.7411) -> (35.3365, -16.916) centre (36.8023, -7.7096) ccw projected
  arc A223 (35.3365, -16.916) -> (36.5863, -17.0535) centre (37.3691, -4.1845) ccw projected
  arc A224 (36.5863, -17.0535) -> (38.3303, -17.0686) centre (37.6027, -0.3965) ccw projected
  arc A225 (38.3303, -17.0686) -> (39.1729, -15.0343) centre (0, 0) ccw projected
  arc A226 (39.1729, -15.0343) -> (37.9291, -13.8118) centre (26.8695, -26.3088) ccw projected
  arc A227 (37.9291, -13.8118) -> (36.9481, -13.0252) centre (29.3828, -23.4651) ccw projected
  arc A228 (36.9481, -13.0252) -> (36.2272, -12.5517) centre (31.4746, -20.5717) ccw projected
  arc A229 (36.2272, -12.5517) -> (36.6861, -11.1393) centre (0, 0) ccw projected
  arc A230 (36.6861, -11.1393) -> (37.5477, -11.1799) centre (37.5552, -1.8575) ccw projected
  arc A231 (37.5477, -11.1799) -> (38.8036, -11.1201) centre (37.5636, 1.7129) ccw projected
  arc A232 (38.8036, -11.1201) -> (40.5285, -10.8623) centre (37.2018, 5.4908) ccw projected
  arc A233 (40.5285, -10.8623) -> (41.0425, -8.7212) centre (0, 0) ccw projected
  arc A234 (41.0425, -8.7212) -> (39.6227, -7.7084) centre (30.6543, -21.7816) ccw projected
  arc A235 (39.6227, -7.7084) -> (38.5308, -7.0849) centre (32.6918, -18.5797) ccw projected
  arc A236 (38.5308, -7.0849) -> (37.7447, -6.73) centre (34.3052, -15.3947) ccw projected
  arc A237 (37.7447, -6.73) -> (37.977, -5.2632) centre (0, 0) ccw projected
  arc A238 (37.977, -5.2632) -> (38.8343, -5.1685) centre (37.3834, 4.0403) ccw projected
  arc A239 (38.8343, -5.1685) -> (40.0655, -4.913) centre (36.8332, 7.568) ccw projected
  arc A240 (40.0655, -4.913) -> (41.7288, -4.3885) centre (35.8848, 11.2428) ccw projected
  arc A241 (41.7288, -4.3885) -> (41.9015, -2.1934) centre (0, 0) ccw projected
  arc A242 (41.9015, -2.1934) -> (40.3408, -1.4151) centre (33.6843, -16.718) ccw projected
  arc A243 (40.3408, -1.4151) -> (39.1647, -0.9701) centre (35.1958, -13.2368) ccw projected
  arc A244 (39.1647, -0.9701) -> (38.3328, -0.7425) centre (36.2911, -9.8386) ccw projected
  arc A245 (38.3328, -0.7425) -> (38.3328, 0.7425) centre (0, 0) ccw projected
  arc A246 (38.3328, 0.7425) -> (39.1647, 0.9701) centre (36.2911, 9.8386) ccw projected
  arc A247 (39.1647, 0.9701) -> (40.3306, 1.4107) centre (35.1958, 13.2368) ccw projected
  arc A248 (40.3306, 1.4107) -> (41.9015, 2.1934) centre (33.6843, 16.718) ccw projected
  arc A249 (41.9015, 2.1934) -> (41.7288, 4.3885) centre (0, 0) ccw projected
  arc A250 (41.7288, 4.3885) -> (40.0655, 4.913) centre (35.8848, -11.2428) ccw projected
  arc A251 (40.0655, 4.913) -> (38.8343, 5.1685) centre (36.8332, -7.568) ccw projected
  arc A252 (38.8343, 5.1685) -> (37.977, 5.2632) centre (37.3834, -4.0403) ccw projected
  arc A253 (37.977, 5.2632) -> (37.7447, 6.73) centre (0, 0) ccw projected
  arc A254 (37.7447, 6.73) -> (38.5308, 7.0849) centre (34.3052, 15.3947) ccw projected
  arc A255 (38.5308, 7.0849) -> (39.6227, 7.7084) centre (32.6918, 18.5797) ccw projected
  arc A256 (39.6227, 7.7084) -> (41.0425, 8.7212) centre (30.6543, 21.7816) ccw projected
  arc A257 (41.0425, 8.7212) -> (40.5285, 10.8623) centre (0, 0) ccw projected
  arc A258 (40.5285, 10.8623) -> (38.8036, 11.1201) centre (37.2018, -5.4908) ccw projected
  arc A259 (38.8036, 11.1201) -> (37.5477, 11.1799) centre (37.5636, -1.7129) ccw projected
  arc A260 (37.5477, 11.1799) -> (36.6861, 11.1393) centre (37.5552, 1.8575) ccw projected
  arc A261 (36.6861, 11.1393) -> (36.2272, 12.5517) centre (0, 0) ccw projected
  arc A262 (36.2272, 12.5517) -> (36.9481, 13.0252) centre (31.4746, 20.5717) ccw projected
  arc A263 (36.9481, 13.0252) -> (37.9207, 13.8045) centre (29.3828, 23.4651) ccw projected
  arc A264 (37.9207, 13.8045) -> (39.1729, 15.0343) centre (26.8695, 26.3088) ccw projected
  arc A265 (39.1729, 15.0343) -> (38.3303, 17.0686) centre (0, 0) ccw projected
  arc A266 (38.3303, 17.0686) -> (36.5863, 17.0535) centre (37.6027, 0.3965) ccw projected
  arc A267 (36.5863, 17.0535) -> (35.3365, 16.916) centre (37.3691, 4.1845) ccw projected
  arc A268 (35.3365, 16.916) -> (34.4919, 16.7411) centre (36.8023, 7.7096) ccw projected
  arc A269 (34.4919, 16.7411) -> (33.8177, 18.0643) centre (0, 0) ccw projected
  arc A270 (33.8177, 18.0643) -> (34.4556, 18.6448) centre (27.869, 25.2421) ccw projected
  arc A271 (34.4556, 18.6448) -> (35.3014, 19.5752) centre (25.3503, 27.7726) ccw projected
  arc A272 (35.3014, 19.5752) -> (36.3388, 20.9772) centre (22.4231, 30.1882) ccw projected
  arc A273 (36.3388, 20.9772) -> (35.1883, 22.8546) centre (0, 0) ccw projected
  arc A274 (35.1883, 22.8546) -> (33.4681, 22.5669) centre (37.0778, 6.2739) ccw projected
  arc A275 (33.4681, 22.5669) -> (32.2552, 22.2356) centre (36.2544, 9.9788) ccw projected
  arc A276 (32.2552, 22.2356) -> (31.4483, 21.9307) centre (35.1431, 13.3718) ccw projected
  arc A277 (31.4483, 21.9307) -> (30.5755, 23.1322) centre (0, 0) ccw projected
  arc A278 (30.5755, 23.1322) -> (31.1147, 23.8053) centre (23.5772, 29.291) ccw projected
  arc A279 (31.1147, 23.8053) -> (31.8046, 24.8565) centre (20.6936, 31.3964) ccw projected
  arc A280 (31.8046, 24.8565) -> (32.6098, 26.4036) centre (17.4245, 33.3243) ccw projected
  arc A281 (32.6098, 26.4036) -> (31.1798, 28.0779) centre (0, 0) ccw projected
  arc A282 (31.1798, 28.0779) -> (29.5259, 27.5246) centre (35.6398, 11.9969) ccw projected
  arc A283 (29.5259, 27.5246) -> (28.3796, 27.0076) centre (34.247, 15.5273) ccw projected
  arc A284 (28.3796, 27.0076) -> (27.6304, 26.5803) centre (32.6187, 18.7048) ccw projected
  arc A285 (27.6304, 26.5803) -> (26.5803, 27.6304) centre (0, 0) ccw projected
  arc A286 (26.5803, 27.6304) -> (27.0076, 28.3796) centre (18.7048, 32.6187) ccw projected
  arc A287 (27.0076, 28.3796) -> (27.5246, 29.5259) centre (15.5273, 34.247) ccw projected
  arc A288 (27.5246, 29.5259) -> (28.0779, 31.1798) centre (11.9969, 35.6398) ccw projected
  arc A289 (28.0779, 31.1798) -> (26.4036, 32.6098) centre (0, 0) ccw projected
  arc A290 (26.4036, 32.6098) -> (24.8565, 31.8046) centre (33.3243, 17.4245) ccw projected
  arc A291 (24.8565, 31.8046) -> (23.8053, 31.1147) centre (31.3964, 20.6936) ccw projected